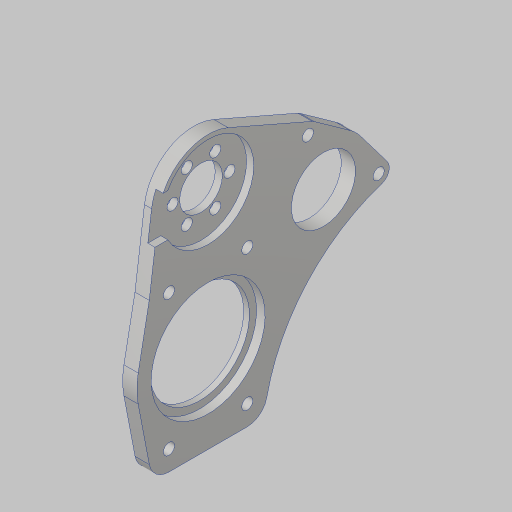
# Autodesk Inventor part: AR-002
Saved by Autodesk Inventor 2023.5 (Build 275446000, 446)
## iProperties
Created: 2025-01-22
Part Number: AR-002
Material: Aluminum 6061
Document SubType Name: Modeling
Designer: slick
Density: 2.7 g/cm^3
Appearance: Aluminum - Flat
Mass: 123.132 g
Surface Area: 216.065 cm^2
Volume: 45.6044 cm^3
Author: slick
Autodesk Inventor part; units mm, degrees
ref_plane "YZ Plane" through (0, 0, 0) normal (1, 0, 0) x (0, 1, 0)
ref_plane "XZ Plane" through (0, 0, 0) normal (0, 1, 0) x (-1, 0, 0)
ref_plane "XY Plane" through (0, 0, 0) normal (0, 0, 1) x (1, 0, 0)
sketch "Sketch1" plane through (0, 0, 0) normal (1, 0, 0) x (0, 1, 0)
  circle A0 centre (0, 0) radius 38.1 construction
  line L0 (27.94, -25.903) -> (27.94, -76.2) construction
  line L1 (27.94, -76.2) -> (-27.94, -76.2) construction
  line L2 (-27.94, -76.2) -> (-27.94, -25.903) construction
  line L3 (-30.1625, -17.4625) -> (30.1625, -17.4625) construction
  line L4 (30.1625, -17.4625) -> (30.1625, 17.4625) construction
  line L5 (30.1625, 17.4625) -> (-30.1625, 17.4625) construction
  line L6 (-30.1625, 17.4625) -> (-30.1625, -17.4625) construction
  line L7 (-30.1625, -17.4625) -> (30.1625, 17.4625) construction
  line L8 (30.1625, -17.4625) -> (-30.1625, 17.4625) construction
  circle A1 centre (30.1625, 17.4625) radius 2.5527 construction
  circle A2 centre (30.1625, -17.4625) radius 2.5527 construction
  circle A3 centre (-30.1625, -17.4625) radius 2.5527 construction
  circle A4 centre (-30.1625, 17.4625) radius 2.5527 construction
  point P0 (0, -76.2)
  dimension "d0" = 76.2
  dimension "d1" = 55.88
  dimension "d2" = 76.2
  dimension "d3" = 60.325
  dimension "d4" = 34.925
  dimension "d5" = 5.1054
  dimension "d6" = 5.1054
  dimension "d7" = 5.1054
  dimension "d8" = 5.1054
  constraints: 18 end point, 5 centre point, 5 coincident, 3 midpoint, 3 perpendicular, 2 parallel, 2 point on circle, 1 horizontal, 1 vertical, 1 vertical alignment
  measures "d0" diameter of A0
  measures "d1" distance of L0.end L1.end
  measures "d2" distance from line of point (0, 0) L1
  measures "d3" distance of L5.end L4.end
  measures "d4" distance of L4.end L3.end
  measures "d5" diameter of A1
  measures "d6" diameter of A2
  measures "d7" diameter of A3
  measures "d8" diameter of A4
sketch "Sketch2" plane through (0, 0, 0) normal (1, 0, 0) x (0, 1, 0)
  line L0 (-30.1625, -17.4625) -> (30.1625, -17.4625) construction
  circle A0 centre (30.1625, -17.4625) radius 2.5527 construction
  circle A1 centre (-30.1625, -17.4625) radius 2.5527 construction
  line L1 (-30.1625, 17.4625) -> (-30.1625, -17.4625) construction
  circle A2 centre (-30.1625, 17.4625) radius 2.5527 construction
  line L2 (30.1625, -17.4625) -> (30.1625, 17.4625) construction
  line L3 (30.1625, -17.4625) -> (-30.1625, 17.4625) construction
  line L4 (30.1625, 17.4625) -> (-30.1625, 17.4625) construction
  line L5 (-30.1625, -17.4625) -> (30.1625, 17.4625) construction
  circle A3 centre (30.1625, 17.4625) radius 2.5527 construction
  circle A4 centre (0, 0) radius 38.1 construction
  line L6 (27.94, -25.903) -> (27.94, -76.2) construction
  line L7 (27.94, -76.2) -> (-27.94, -76.2) construction
  line L8 (-27.94, -76.2) -> (-27.94, -25.903) construction
  circle A5 centre (60.325, 0) radius 12.7 construction
  circle A6 centre (35.56, -51.3927) radius 14.2875
  circle A7 centre (35.56, -51.3927) radius 25.4 construction
  circle A8 centre (60.325, 0) radius 9.525
  circle A9 centre (60.325, 0) radius 22.225 construction
  circle A10 centre (30.1625, 17.4625) radius 8.9027 construction
  circle A11 centre (30.1625, -17.4625) radius 8.9027 construction
  circle A12 centre (-30.1625, -17.4625) radius 8.9027 construction
  circle A13 centre (-30.1625, 17.4625) radius 8.9027 construction
  line L9 (63.2628, 22.03) -> (31.3393, 26.2871)
  line L10 (-39.0652, 17.4625) -> (-39.0652, -17.4625)
  arc A14 (80.7011, -8.875) -> (63.2628, 22.03) centre (60.325, 0) ccw
  arc A15 (31.3393, 26.2871) -> (31.8447, 26.2048) centre (30.1625, 17.4625) ccw
  arc A16 (-31.8447, 26.2048) -> (-39.0652, 17.4625) centre (-30.1625, 17.4625) ccw
  arc A17 (-39.0652, -17.4625) -> (-32.0045, -26.1726) centre (-30.1625, -17.4625) ccw
  circle A18 centre (35.56, -51.3927) radius 25.4 construction
  circle A19 centre (17.3498, -33.6855) radius 4.7625 construction
  circle A20 centre (29.3302, -76.0169) radius 4.7625 construction
  circle A21 centre (60.0001, -44.4759) radius 4.7625 construction
  circle A22 centre (0, 0) radius 25.4
  circle A23 centre (0, 0) radius 31.75 construction
  line L11 (31.8447, 26.2048) -> (5.9993, 31.178)
  line L12 (-5.9993, 31.178) -> (-31.8447, 26.2048)
  arc A24 (5.9993, 31.178) -> (-5.9993, 31.178) centre (0, 0) ccw
  circle A25 centre (35.56, -51.3927) radius 29.9974 construction
  circle A26 centre (35.56, -51.3927) radius 20.6375 construction
  arc A27 (24.7948, -77.4703) -> (-32.0045, -26.1726) centre (-47.7704, -100.7237) ccw
  arc A28 (24.7948, -77.4703) -> (32.2043, -79.8144) centre (29.3302, -76.0169) ccw
  circle A29 centre (35.56, -51.3927) radius 7.62 construction
  line L13 (80.7011, -8.875) -> (64.3664, -46.3776)
  line L14 (63.8765, -47.2425) -> (52.3581, -63.3816)
  line L15 (32.2043, -79.8144) -> (48.0145, -67.8485)
  arc A30 (48.0145, -67.8485) -> (52.3581, -63.3816) centre (35.56, -51.3927) ccw
  arc A31 (63.8765, -47.2425) -> (64.3664, -46.3776) centre (60.0001, -44.4759) ccw
  point P0 (0, -76.2)
  point P1 (71.3235, -6.35)
  point P2 (71.3235, 6.35)
  point P3 (60.325, 12.7)
  point P4 (49.3265, 6.35)
  point P5 (49.3265, -6.35)
  point P6 (60.325, -12.7)
  point P7 (31.5932, 26.2532)
  dimension "d9" = 25.4
  dimension "d76" = 50.8
  dimension "d14" = 360
  dimension "d16" = 28.575
  dimension "d17" = 57.0484
  dimension "d19" = 50.8
  dimension "d20" = 19.05
  dimension "d23" = 6.35
  dimension "d43" = 360
  dimension "d45" = 9.525
  dimension "d46" = 9.525
  dimension "d47" = 9.525
  dimension "d56" = 50.8
  dimension "d57" = 6.35
  dimension "d58" = 44.45
  dimension "d60" = 76.2
  dimension "d65" = 59.9948
  dimension "d66" = 6.35
  dimension "d67" = 76.2
  dimension "d75" = 15.24
  constraints: 35 point on circle, 25 centre point, 19 coincident, 19 tangent, 14 end point, 4 equal radius, 2 midpoint, 1 vertical alignment, 17 other
  measures "d16" diameter of A6
  measures "d17" distance of A6.centre A9.centre
  measures "d19" diameter of A7
  measures "d20" diameter of A8
  measures "d23" radial gap between concentric circles of A3 A10
  measures "d45" diameter of A19
  measures "d46" diameter of A20
  measures "d47" diameter of A21
  measures "d56" diameter of A22
  measures "d57" radial gap between concentric circles of A22 A23
  measures "d58" diameter of A9
  measures "d60" distance from line of L7 A9.centre
  measures "d65" diameter of A25
  measures "d66" radial gap between concentric circles of A6 A26
  measures "d67" radius of A27
  measures "d75" diameter of A29
extrude "Extrusion1" add sketch "Sketch2" along normal blind 6.35 contours L11 A15 L9 | A14 L13 A31 L14 A30 L15 A28 A27 A17 L10 A16 L12 A24 L11 L9
hole "Motor Mount Holes" at (0, -30.1625, -17.4625) at (0, 30.1625, -17.4625) at (0, -30.1625, 17.4625) at (0, 30.1625, 17.4625) at (0, 0, -76.2) at (0, 71.3235, -6.35) at (0, 71.3235, 6.35) at (0, 60.325, 12.7) at (0, 49.3265, 6.35) at (0, 49.3265, -6.35) at (0, 60.325, -12.7) direction (1, 0, 0) diameter 4.9784 end through all clearance for "Flat Head Machine Screw (82)" size "#10" standard "Ansi Unified Screw Threads"
hole "Hole3" at (0, 60.0001, -44.4759) at (0, 29.3302, -76.0169) direction (1, 0, 0) diameter 4.9784 end through all clearance for "Flat Head Machine Screw (82)" size "#10" standard "Ansi Unified Screw Threads"
sketch "Sketch3" plane through (6.35, 0, 0) normal (1, 0, 0) x (0, 0, -1)
  circle A0 centre (0, 60.325) radius 9.525 projected
  circle A1 centre (0, 60.325) radius 20.32
  point P0 (0, 0)
  dimension "d61" = 40.64
  constraints: 1 centre point, 1 coincident
  measures "d61" diameter of A1
extrude "Extrusion2" cut sketch "Sketch3" against normal blind 3.175
sketch "Sketch4" plane through (6.35, 0, 0) normal (1, 0, 0) x (0, 0, -1)
  circle A0 centre (0, 60.325) radius 20.32 projected
  circle A1 centre (44.4759, 60.0001) radius 2.4892 projected
  circle A2 centre (76.0169, 29.3302) radius 2.4892 projected
  circle A3 centre (-17.4625, 30.1625) radius 2.4892 projected
  circle A4 centre (17.4625, 30.1625) radius 2.4892 projected
  circle A5 centre (17.4625, -30.1625) radius 2.4892 projected
  circle A6 centre (-17.4625, -30.1625) radius 2.4892 projected
  circle A7 centre (51.3927, 35.56) radius 14.2875 projected
  circle A8 centre (0, 0) radius 25.4 projected
  arc A9 (77.4703, 24.7948) -> (26.1726, -32.0045) centre (100.7237, -47.7704) ccw projected
  arc A10 (17.4625, -39.0652) -> (26.1726, -32.0045) centre (17.4625, -30.1625) ccw projected
  line L0 (17.4625, -39.0652) -> (-17.4625, -39.0652) projected
  arc A11 (-26.2048, -31.8447) -> (-17.4625, -39.0652) centre (-17.4625, -30.1625) ccw projected
  line L1 (-26.2048, -31.8447) -> (-31.178, -5.9993) projected
  arc A12 (-31.178, 5.9993) -> (-31.178, -5.9993) centre (0, 0) ccw projected
  line L2 (-31.178, 5.9993) -> (-26.2532, 31.5932) projected
  line L3 (-26.2532, 31.5932) -> (-22.03, 63.2628) projected
  arc A13 (8.875, 80.7011) -> (-22.03, 63.2628) centre (0, 60.325) ccw projected
  line L4 (-20.0805, 69.85) -> (-17.9493, 69.85)
  circle A14 centre (0, 60.325) radius 20.32 projected
  line L5 (-22.03, 63.2628) -> (-26.2532, 31.5932) projected
  line L6 (-23.6919, 50.8) -> (-17.9493, 50.8)
  arc A15 (8.875, 80.7011) -> (-22.03, 63.2628) centre (0, 60.325) ccw projected
  line L7 (8.875, 80.7011) -> (46.3776, 64.3664) projected
  arc A16 (47.2425, 63.8765) -> (46.3776, 64.3664) centre (44.4759, 60.0001) ccw projected
  line L8 (47.2425, 63.8765) -> (63.3816, 52.3581) projected
  arc A17 (67.8485, 48.0145) -> (63.3816, 52.3581) centre (51.3927, 35.56) ccw projected
  line L9 (67.8485, 48.0145) -> (79.8144, 32.2043) projected
  arc A18 (77.4703, 24.7948) -> (79.8144, 32.2043) centre (76.0169, 29.3302) ccw projected
  point P0 (5.7277, 81.7993)
  point P1 (-20.8206, 50.8)
  point P2 (-19.0149, 69.85)
  dimension "d68" = 19.05
  dimension "d69" = 9.525
  constraints: 4 end point, 2 midpoint, 1 horizontal, 1 parallel, 1 point on circle, 1 point on line, 4 other
  measures "d68" vertical distance of point (-20.821, 50.8) point (-19.015, 69.85)
  measures "d69" vertical distance of point (0, 60.325) point (-19.015, 69.85)
extrude "Extrusion3" cut sketch "Sketch4" against normal blind 3.175 contours A0 L6 L3 A13 L4
sketch "Sketch5" plane through (0, 0, 0) normal (-1, 0, 0) x (0, 0, 1)
  circle A0 centre (0, 0) radius 22.225
  circle A1 centre (0, 0) radius 25.4 projected
  dimension "d72" = 44.45
  constraints: 1 centre point, 1 coincident
  measures "d72" diameter of A0
extrude "Extrusion4" add sketch "Sketch5" against normal blind 2.54
body "Solid1"
